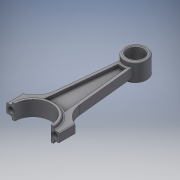
# Autodesk Inventor part: BIELA PART 2
Saved by Autodesk Inventor 2019.3 (Build 233278000, 278)
## iProperties
Created: 2017-10-06
Part Number: BIELA PART 2
Material: Generic
Document SubType Name: Modeling
Designer: Usuario
Density: 1 g/cm^3
Appearance: Default
Author: Usuario
Autodesk Inventor part; units mm, degrees
ref_plane "XZ Plane" through (0, 0, 0) normal (0, 1, 0) x (-1, 0, 0)
ref_plane "XY Plane" through (0, 0, 0) normal (0, 0, 1) x (1, 0, 0)
sketch "Sketch1" plane through (0, 0, 0) normal (0, 0, 1) x (1, 0, 0)
  circle A0 centre (0, 0) radius 15
  circle A1 centre (0, 0) radius 10.5
  dimension "d0" = 30
  dimension "d1" = 21
  constraints: 2 centre point, 2 coincident
  measures "d0" diameter of A0
  measures "d1" diameter of A1
extrude "Extrusion1" add sketch "Sketch1" along normal mid plane 25
sketch "Sketch2" plane through (0, 0, 0) normal (0, 0, 1) x (1, 0, 0)
  arc A0 (27.5, -135) -> (-27.5, -135) centre (0, -135) ccw
  arc A1 (22.5, -135) -> (-22.5, -135) centre (0, -135) ccw
  line L0 (27.5, -135) -> (22.5, -135)
  line L1 (-22.5, -135) -> (-27.5, -135)
  point P0 (0, 0)
  dimension "d8" = 55
  dimension "d9" = 45
  dimension "d10" = 135
  constraints: 4 end point, 4 point on circle, 2 centre point, 1 coincident
  measures "d8" diameter of A0
  measures "d9" diameter of A1
  measures "d10" distance of point (0, 0) A0.centre
extrude "Extrusion2" add sketch "Sketch2" along normal mid plane 20
sketch "Sketch3" plane through (0, 0, 0) normal (0, 0, 1) x (1, 0, 0)
  circle A0 centre (0, 0) radius 15 projected
  arc A1 (27.5, -135) -> (-27.5, -135) centre (0, -135) ccw projected
  line L0 (8, -12.6886) -> (18.5, -114.653)
  line L1 (0, 0) -> (0, -135)
  line L2 (-8, -12.6886) -> (-18.5, -114.653)
  arc A2 (18.5, -114.653) -> (-18.5, -114.653) centre (0, -135) ccw
  arc A3 (-8, -12.6886) -> (8, -12.6886) centre (0, 0) ccw
  dimension "d14" = 18.5
  dimension "d15" = 8
  constraints: 6 end point, 5 point on circle, 2 centre point, 2 coincident, 2 symmetric about line, 1 vertical, 2 other
  measures "d14" horizontal distance of L1.end L0.end
  measures "d15" horizontal distance of L0.start point (0, 0)
extrude "Extrusion3" add sketch "Sketch3" along normal mid plane 12 contours A0 L1 A1 L2 | L0 A1 L1 A0
sketch "Sketch4" plane through (0, 0, 6) normal (0, 0, 1) x (1, 0, 0)
  line L0 (-8, -12.6886) -> (-18.5, -114.653) projected
  line L1 (18.5, -114.653) -> (8, -12.6886) projected
  line L2 (18.5, -114.653) -> (8, -12.6886) projected
  arc A0 (-8, -12.6886) -> (8, -12.6886) centre (0, 0) ccw projected
  line L3 (-8, -12.6886) -> (-18.5, -114.653) projected
  arc A1 (18.5, -114.653) -> (-18.5, -114.653) centre (0, -135) ccw projected
  line L4 (-14.2222, -107.4368) -> (-4.9947, -17.8297)
  arc A2 (-4.9947, -17.8297) -> (4.9947, -17.8297) centre (0, 0) ccw
  line L5 (4.9947, -17.8297) -> (14.2222, -107.4368)
  arc A3 (14.2222, -107.4368) -> (-14.2222, -107.4368) centre (0, -135) ccw
  dimension "d18" = 3.5161
  constraints: 4 end point, 4 point on circle, 2 centre point, 3 other
  measures "d18" radial gap between concentric circles of A1 A3
extrude "Extrusion4" cut sketch "Sketch4" against normal blind 5 contours L4 A2 L5 A3
mirror "Mirror1" about plane through (0, 0, 0) normal (0, 0, 1) of "Extrusion4"
sketch "Sketch5" plane through (0, 0, 0) normal (0, 0, 1) x (1, 0, 0)
  point P0 (0, 0)
ref_plane "Work Plane1" through (-35, 0, 0) normal (1, 0, 0) x (0, 1, 0)
sketch "Sketch6" plane through (-35, 0, 0) normal (1, 0, 0) x (0, 1, 0)
  line L0 (-114.653, -6) -> (-12.6886, -6) projected
  line L1 (-135, -10) -> (-135, 10) projected
  line L2 (-114.653, -6) -> (-135, -6)
  line L3 (-135, -6) -> (-135, 6)
  line L4 (-135, 6) -> (-114.653, 6)
  line L5 (-114.653, 6) -> (-114.653, -6)
  line L6 (-12.6886, 6) -> (-114.653, 6) projected
  point P0 (0, 0)
  constraints: 8 end point, 2 parallel, 1 horizontal, 1 perpendicular, 1 point on line
extrude "Extrusion5" add sketch "Sketch6" along normal up to next
mirror "Mirror2" about plane through (0, 0, 0) normal (1, 0, 0) of "Extrusion5"
fillet "Fillet1" radius 30 2 edges at (18.5, -114.653, 0) (-18.5, -114.653, 0)
sketch "Sketch7" plane through (-27.5, -135, -10) normal (0, -1, 0) x (1, 0, 0)
  circle A0 centre (-1.25, 10) radius 2.65
  line L0 (-7.5, 16) -> (-7.5, 4) projected
  point P0 (27.5, 10)
  dimension "d25" = 5.3
  dimension "d26" = 6.25
  constraints: 1 centre point, 1 horizontal alignment
  measures "d25" diameter of A0
  measures "d26" distance from line of L0 A0.centre
extrude "Extrusion6" cut sketch "Sketch7" against normal blind 20
sketch "Sketch8" plane through (-27.5, -135, -10) normal (0, -1, 0) x (1, 0, 0)
  circle A0 centre (-1.25, 10) radius 2.65 projected
  line L0 (5, 20) -> (5, 0) projected
  circle A1 centre (-1.25, 10) radius 2.65 projected
  point P0 (27.5, 10)
mirror "Mirror4" about plane through (0, 0, 0) normal (1, 0, 0) of "Extrusion6"
chamfer "Chamfer1" distance 1 angle 45 2 edges at (-10.5, 0, 12.5) (-10.5, 0, -12.5)
fillet "Fillet2" radius 2 1 edges at (0, -107.5, 6)
fillet "Fillet3" radius 2 1 edges at (0, -107.5, -6)
fillet "Fillet4" radius 1 2 edges at (0, -107.5, -10) (0, -107.5, 10)
fillet "Fillet5" radius 1.5 4 edges at (-35, -124.8265, -6) (-35, -124.8265, 6) (35, -124.8265, -6) (35, -124.8265, 6)
fillet "Fillet6" radius 2 2 edges at (-15, 0, -12.5) (-15, 0, 12.5)
fillet "Fillet7" radius 1 4 edges at (0, -103.9839, -1) (9.6084, -62.6333, -1) (-9.6084, -62.6333, -1) (0, -18.5161, -1)
fillet "Fillet8" radius 1 4 edges at (0, -103.9839, 1) (-9.6084, -62.6333, 1) (9.6084, -62.6333, 1) (0, -18.5161, 1)
fillet "Fillet9" radius 1 2 edges at (0, -112.5, 10) (0, -112.5, -10)
scale "Scale6" factors (0.24, 0.24, 0.24) then translate (0, 0, 0) bodies 1
sketch "Sketch10" plane through (6.6, -32.4, -2.16) normal (0, -1, 0) x (1, 0, 0)
  circle A0 centre (-13.5, 2.16) radius 0.636 projected
  circle A1 centre (-13.5, 2.16) radius 1
  circle A2 centre (0.3, 2.16) radius 0.636 projected
  circle A3 centre (0.3, 2.16) radius 1
  point P0 (-6.6, 2.16)
  dimension "d62" = 2
  dimension "d63" = 2
  constraints: 2 centre point, 2 coincident
  measures "d62" diameter of A1
  measures "d63" diameter of A3
extrude "Extrusion8" cut sketch "Sketch10" against normal blind 10 contours A0 | A1 | A2 | A3
sketch "Sketch12" plane through (0, -32.4, 2.4) normal (0, 0, 1) x (1, 0, 0)
  circle A0 centre (0, 0) radius 5.75
  point P0 (0, 32.4)
  dimension "d70" = 11.5
  constraints: 1 centre point
  measures "d70" diameter of A0
extrude "Extrusion10" cut sketch "Sketch12" against normal through all
body "Solid1"
